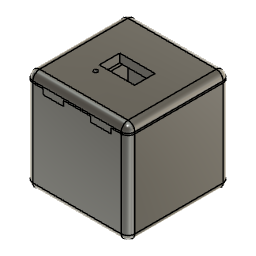
aashish (Autodesk Fusion 360 design; units mm, degrees)
Autodesk Fusion 360 part; units mm, degrees
note: some values were not read from the file. Chosen so that the rebuilt part matches the saved one: which face or edge a step refers to. Set by a fixed rule: which sketch regions a step uses.
sketch "Sketch1" plane through (0, 0, 0) normal (0, 0, 1) x (1, 0, 0)
  line L0 (0, 0) -> (30, 0)
  line L1 (30, 0) -> (30, 30)
  line L2 (30, 30) -> (0, 30)
  line L3 (0, 30) -> (0, 0)
  dimension "d1" = 30
  dimension "d2" = 30
  constraint horizontal L0
  constraint vertical L1
  constraint horizontal L2
  constraint vertical L3
  constraint coincident L0.start L3.end
  measures "d1" distance of L0.start L0.end
  measures "d2" distance of L0.start L2.end
extrude "Extrude1" add sketch "Sketch1" along normal blind 30 makes body 1
fillet "Fillet1" radius 2 12 edges at (0, 30, 15) (0, 0, 15) (0, 15, 0) (0, 15, 30) (30, 30, 15) (15, 30, 0) (15, 30, 30) (30, 0, 15) (30, 15, 0) (30, 15, 30) (15, 0, 0) (15, 0, 30) on bodies 1
shell "Shell1" thickness 2.5 removed faces 0 bodies 1
ref_plane "WorkPlane1" through (15, 15, 27.5) normal (0, 0, 1) x (1, 0, 0)
split "Split1" by plane through (15, 15, 27.5) normal (0, 0, 1) bodies 1 makes body 2 at (10.6667, 19.3333, 30)
sketch "Sketch2" plane through (0, 0, 30) normal (0, 0, 1) x (-1, 0, 0)
  line L0 (-2, -2) -> (-28, -2)
  line L1 (-28, -2) -> (-28, -28)
  line L2 (-28, -28) -> (-2, -28)
  line L3 (-2, -28) -> (-2, -2)
  line L4 (-22.5, -22.5) -> (-22.5, -7.5)
  line L5 (-7.5, -7.5) -> (-7.5, -22.5)
  line L6 (-22.5, -7.5) -> (-7.5, -7.5)
  line L7 (-7.5, -22.5) -> (-22.5, -22.5)
  line L8 (-9.7162, -21.0598) -> (-9.038, -21.0598)
  line L9 (-8.088, -20.4599) -> (-8.078, -21.94)
  line L10 (-9.978, -20.6) -> (-9.978, -21.94)
  line L11 (-8.078, -21.94) -> (-9.978, -21.94)
  line L12 (-9.9879, -18.2099) -> (-9.638, -17.8599)
  line L13 (-9.988, -18.2099) -> (-9.9879, -18.2099)
  line L14 (-8.088, -18.2099) -> (-8.4379, -17.8599)
  line L15 (-8.088, -18.2099) -> (-8.088, -18.2099)
  line L16 (-8.088, -19.4599) -> (-8.088, -18.2099)
  line L17 (-9.988, -19.4599) -> (-9.988, -18.2099)
  line L18 (-8.4379, -17.8599) -> (-9.638, -17.8599)
  line L19 (-8.538, -20.26) -> (-9.538, -20.26)
  line L20 (-9.043, -20.26) -> (-9.043, -19.76)
  line L21 (-8.939, -9.9419) -> (-8.939, -9.604)
  line L22 (-10.7891, -11.2729) -> (-9.8703, -11.2729)
  line L23 (-12.5892, -8.7417) -> (-12.5892, -8.2728)
  line L24 (-12.5892, -8.2728) -> (-12.5892, -8.7417)
  line L25 (-12.5892, -10.8042) -> (-12.5892, -11.2728)
  line L26 (-12.5892, -11.2728) -> (-12.5892, -10.8042)
  line L27 (-12.5892, -8.2728) -> (-9.8703, -8.2728)
  line L28 (-12.5892, -8.7417) -> (-12.5892, -8.2728)
  line L29 (-12.5892, -11.2728) -> (-12.5892, -10.8042)
  line L30 (-10.7891, -11.2728) -> (-12.5892, -11.2728)
  line L31 (-10.7891, -8.2728) -> (-12.5892, -8.2728)
  line L32 (-10.943, -19.579) -> (-10.943, -22.0936)
  line L33 (-18.563, -19.579) -> (-13.483, -19.579)
  line L34 (-13.483, -19.579) -> (-10.943, -19.579)
  line L35 (-10.943, -22.0936) -> (-18.563, -22.0936)
  line L36 (-18.563, -22.0936) -> (-18.563, -19.579)
  line L37 (-8.338, -20.96) -> (-8.338, -21.16)
  line L38 (-8.338, -21.16) -> (-9.738, -21.16)
  line L39 (-9.738, -20.96) -> (-8.338, -20.96)
  line L40 (-9.738, -21.16) -> (-9.738, -20.96)
  line L41 (-9.1322, -21.5946) -> (-8.9822, -21.5946)
  line L42 (-8.9822, -20.5946) -> (-9.1322, -20.5946)
  line L43 (-9.1322, -20.5946) -> (-9.1322, -21.5946)
  line L44 (-8.9822, -21.5946) -> (-8.9822, -20.5946)
  line L45 (-9.6799, -17.8799) -> (-20.0798, -17.8799)
  line L46 (-20.0798, -17.8799) -> (-20.0798, -11.8798)
  line L47 (-20.0798, -11.8798) -> (-9.6799, -11.8798)
  line L48 (-9.6799, -11.8798) -> (-9.6799, -17.8799)
  circle A0 centre (-10.7139, -9.7727) radius 0.5752
extrude "Extrude2" cut sketch "Sketch2" against normal blind 2.5 contours L45 L46 L47 L48 | A0 bodies 2
ref_plane "WorkPlane3" through (15, 15, 14.75) normal (0, 1, 0) x (-1, 0, 0)
ref_plane "WorkPlane4" through (15, 15, 14.75) normal (-1, 0, 0) x (0, -1, 0)
sketch "Sketch9" plane through (0, 0, 27.5) normal (0, 0, -1) x (1, 0, 0)
  line L0 (20.0798, -11.8798) -> (20.0798, -17.8799)
  line L1 (20.0798, -17.8799) -> (9.6799, -17.8799)
  line L2 (9.6799, -17.8799) -> (9.6799, -11.8798)
  line L3 (9.6799, -11.8798) -> (20.0798, -11.8798)
  circle A0 centre (10.7139, -9.7727) radius 0.5752
  arc A1 (0, -28) -> (2, -30) centre (2, -28) ccw
  line L4 (2, -30) -> (28, -30)
  arc A2 (28, -30) -> (30, -28) centre (28, -28) ccw
  line L5 (30, -28) -> (30, -2)
  arc A3 (30, -2) -> (28, 0) centre (28, -2) ccw
  line L6 (28, 0) -> (2, 0)
  arc A4 (2, 0) -> (0, -2) centre (2, -2) ccw
  line L7 (0, -2) -> (0, -28)
  line L8 (22.5, -22.5) -> (7.5, -22.5)
  line L9 (7.5, -22.5) -> (7.5, -7.5)
  line L10 (7.5, -7.5) -> (22.5, -7.5)
  line L11 (22.5, -7.5) -> (22.5, -22.5)
  line L12 (5.5, -5.5) -> (24.5, -5.5)
  line L13 (24.5, -5.5) -> (24.5, -24.5)
  line L14 (24.5, -24.5) -> (5.5, -24.5)
  line L15 (5.5, -24.5) -> (5.5, -5.5)
  line L16 (17.5, -24.5) -> (12.5, -24.5)
  line L17 (12.5, -24.5) -> (12.5, -22.5)
  line L18 (12.5, -22.5) -> (17.5, -22.5)
  line L19 (17.5, -22.5) -> (17.5, -24.5)
  line L20 (17.5, -5.5) -> (12.5, -5.5)
  line L21 (12.5, -5.5) -> (12.5, -7.5)
  line L22 (12.5, -7.5) -> (17.5, -7.5)
  line L23 (17.5, -7.5) -> (17.5, -5.5)
  dimension "d105" = 7.5
  dimension "d106" = 7.5
  dimension "d107" = 15
  dimension "d108" = 15
  dimension "d109" = -2
  dimension "d110" = 5
  dimension "d111" = 7
  constraint horizontal L8
  constraint vertical L9
  constraint horizontal L10
  constraint vertical L11
  constraint horizontal L16
  constraint vertical L17
  constraint horizontal L18
  constraint vertical L19
  constraint coincident L8 L17.end
  constraint coincident L14 L16.start
  constraint horizontal L20
  constraint vertical L21
  constraint horizontal L22
  constraint vertical L23
  constraint coincident L10 L21.end
  constraint coincident L12 L20.start
  constraint collinear L19 L23
  constraint collinear L17 L21
  measures "d105" distance of L6 L10
  measures "d106" distance of L7 L9
  measures "d107" distance of L9.end L10.end
  measures "d108" distance of L8.end L9.end
  measures "d110" distance of L21 L23
  measures "d111" distance of L15 L21
extrude "Extrude9" add sketch "Sketch9" along normal blind 3 contours L8 L10 L11 L12 L13 L14 L19 L23 | L8 L9 L10 L12 L14 L15 L17 L21 bodies 2
sketch "Sketch8" plane through (15, 0, 0) normal (-1, 0, 0) x (0, -1, 0)
  line L0 (0, 27.5) -> (-0.9, 27.5)
  line L1 (-2, 27.5) -> (-28, 27.5)
  line L2 (0, 27.5) -> (0, 28)
  line L3 (0, 27.5) -> (0, 26)
  line L4 (0, 26) -> (-0.9, 26)
  line L5 (-1.25, 26.55) -> (-0.9, 26)
  line L6 (-1.25, 26.55) -> (-0.9, 27.1)
  line L7 (-0.9, 27.1) -> (-0.9, 27.5)
  dimension "d114" = 0.9
  dimension "d116" = 1.5
  dimension "d148" = 0.35
  dimension "d149" = 0.9
  dimension "d150" = 0.4
  constraint collinear L0 L1
  constraint coincident L0.start L2.start
  constraint perpendicular L0 L3
  constraint perpendicular L3 L4
  constraint equal L5 L6
  constraint perpendicular L0 L7
  measures "d114" distance of L3.end L4.end
  measures "d116" distance of L0.start L3.end
  measures "d148" horizontal distance of L4.end L5.start
  measures "d149" distance of L0.start L0.end
  measures "d150" distance of L0.end L6.end
extrude "Extrude10" add sketch "Sketch8" along normal blind 6 from surface at 4 bodies 2
mirror "Mirror7" about plane through (15, 15, 14.75) normal (-1, 0, 0) of "Extrude10"
mirror "Mirror8" about plane through (15, 15, 14.75) normal (0, 1, 0) of "Extrude10", "Mirror7"
combine "Combine5" operation cut target body 1 tool bodies 2 keep tools
sketch "Sketch12" plane through (25, 0, 0) normal (-1, 0, 0) x (0, -1, 0)
  line L0 (-1.25, 26.55) -> (-0.9, 26)
  line L1 (-0.9, 26) -> (0, 26)
  line L2 (0, 26) -> (0, 27.5)
  line L3 (0, 27.5) -> (-0.9, 27.5)
  line L4 (-0.9, 27.5) -> (-0.9, 27.1)
  line L5 (-0.9, 27.1) -> (-1.25, 26.55)
  line L6 (-1.1531, 27.2611) -> (-1.6056, 26.55)
  line L7 (-1.6056, 26.55) -> (-1.1531, 25.8389)
  line L8 (0, 26) -> (-1.2556, 26)
  line L9 (-1.1531, 27.2611) -> (-1.001, 27.5)
  line L10 (-1.001, 27.5) -> (0, 27.5)
  line L11 (0, 26) -> (0, 27.5)
  line L12 (-1.001, 27.5) -> (0, 27.5)
  dimension "d151" = 0.3
  constraint coincident L1.end L2.start
  constraint coincident L7 L8.end
  constraint perpendicular L2 L8
  constraint parallel L6 L9
  constraint coincident L2.end L3.start
  constraint perpendicular L2 L10
extrude "Extrude13" cut sketch "Sketch12" along normal blind 6 contours L0 L4 L5 L6 L7 L8 L9 L10 L12 bodies 1
mirror "Mirror11" about plane through (15, 15, 14.75) normal (0, 1, 0) of "Extrude13"
mirror "Mirror12" about plane through (15, 15, 14.75) normal (-1, 0, 0) of "Extrude13", "Mirror11"
named bodies: "Enclosure", "Lid"
